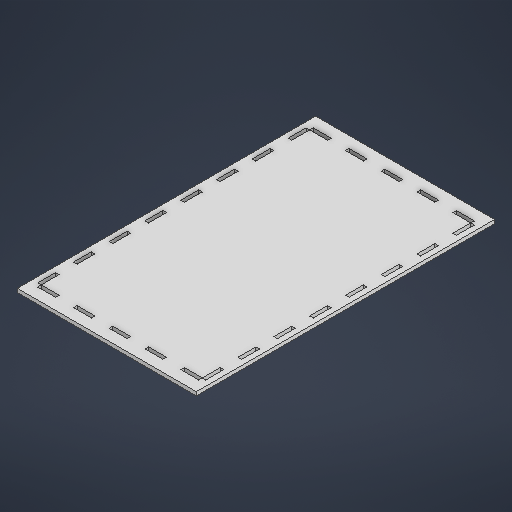
# Autodesk Inventor part: base
Saved by Autodesk Inventor 2026 (Build 300175000, 175)
## iProperties
Created: 2026-04-21
Part Number: base
Material: Generic
Document SubType Name: Modeling
Designer: juana
Density: 1 g/cm^3
Appearance: Default
Author: juana
Autodesk Inventor part; units mm, degrees
ref_plane "YZ Plane" through (0, 0, 0) normal (1, 0, 0) x (0, 1, 0)
ref_plane "XZ Plane" through (0, 0, 0) normal (0, 1, 0) x (-1, 0, 0)
ref_plane "XY Plane" through (0, 0, 0) normal (0, 0, 1) x (1, 0, 0)
sketch "Sketch1" plane through (0, 0, 0) normal (0, 1, 0) x (-1, 0, 0)
  line L0 (0, 0) -> (-150, 0)
  line L1 (-150, 0) -> (-150, -250)
  line L2 (-150, -250) -> (0, -250)
  line L3 (0, -250) -> (0, 0)
  dimension "d0" = 250
  dimension "d1" = 150
  constraints: 8 end point, 2 parallel, 1 coincident, 1 horizontal, 1 horizontal alignment, 1 perpendicular
  measures "d0" distance of L2.end L0.start
  measures "d1" distance of L0.start L0.end
extrude "Extrusion1" add sketch "Sketch1" along normal blind 3.05
sketch "Sketch2" plane through (0, 3.05, 0) normal (0, 1, 0) x (1, 0, 0)
  line L0 (7.5, 9.5) -> (22.5, 9.5)
  line L1 (22.5, 9.5) -> (22.5, 12.5)
  line L2 (22.5, 12.5) -> (7.5, 12.5)
  line L3 (7.5, 12.5) -> (7.5, 9.5)
  line L4 (7.5, 12.5) -> (142.5, 12.5) construction
  line L5 (142.5, 12.5) -> (142.5, 237.5) construction
  line L6 (142.5, 237.5) -> (7.5, 237.5) construction
  line L7 (7.5, 237.5) -> (7.5, 12.5) construction
  line L8 (0, 0) -> (150, 0) projected
  line L9 (0, 250) -> (0, 0) projected
  line L10 (37.5, 12.5) -> (37.5, 9.5)
  line L11 (37.5, 9.5) -> (52.5, 9.5)
  line L12 (52.5, 12.5) -> (37.5, 12.5)
  line L13 (52.5, 9.5) -> (52.5, 12.5)
  line L14 (67.5, 12.5) -> (67.5, 9.5)
  line L15 (67.5, 9.5) -> (82.5, 9.5)
  line L16 (82.5, 12.5) -> (67.5, 12.5)
  line L17 (82.5, 9.5) -> (82.5, 12.5)
  line L18 (97.5, 12.5) -> (97.5, 9.5)
  line L19 (97.5, 9.5) -> (112.5, 9.5)
  line L20 (112.5, 12.5) -> (97.5, 12.5)
  line L21 (112.5, 9.5) -> (112.5, 12.5)
  line L22 (127.5, 12.5) -> (127.5, 9.5)
  line L23 (127.5, 9.5) -> (142.5, 9.5)
  line L24 (142.5, 12.5) -> (127.5, 12.5)
  line L25 (142.5, 9.5) -> (142.5, 12.5)
  line L26 (7.5, 240.5) -> (7.5, 237.5)
  line L27 (7.5, 237.5) -> (22.5, 237.5)
  line L28 (22.5, 240.5) -> (7.5, 240.5)
  line L29 (22.5, 237.5) -> (22.5, 240.5)
  line L30 (37.5, 240.5) -> (37.5, 237.5)
  line L31 (37.5, 237.5) -> (52.5, 237.5)
  line L32 (52.5, 240.5) -> (37.5, 240.5)
  line L33 (52.5, 237.5) -> (52.5, 240.5)
  line L34 (67.5, 240.5) -> (67.5, 237.5)
  line L35 (67.5, 237.5) -> (82.5, 237.5)
  line L36 (82.5, 240.5) -> (67.5, 240.5)
  line L37 (82.5, 237.5) -> (82.5, 240.5)
  line L38 (97.5, 240.5) -> (97.5, 237.5)
  line L39 (97.5, 237.5) -> (112.5, 237.5)
  line L40 (112.5, 240.5) -> (97.5, 240.5)
  line L41 (112.5, 237.5) -> (112.5, 240.5)
  line L42 (127.5, 240.5) -> (127.5, 237.5)
  line L43 (127.5, 237.5) -> (142.5, 237.5)
  line L44 (142.5, 240.5) -> (127.5, 240.5)
  line L45 (142.5, 237.5) -> (142.5, 240.5)
  line L46 (142.5, 12.5) -> (145.5, 12.5)
  line L47 (145.5, 12.5) -> (145.5, 27.5)
  line L48 (145.5, 27.5) -> (142.5, 27.5)
  line L49 (142.5, 27.5) -> (142.5, 12.5)
  line L50 (142.5, 57.5) -> (142.5, 42.5)
  line L51 (142.5, 42.5) -> (145.5, 42.5)
  line L52 (145.5, 57.5) -> (142.5, 57.5)
  line L53 (145.5, 42.5) -> (145.5, 57.5)
  line L54 (142.5, 87.5) -> (142.5, 72.5)
  line L55 (142.5, 72.5) -> (145.5, 72.5)
  line L56 (145.5, 87.5) -> (142.5, 87.5)
  line L57 (145.5, 72.5) -> (145.5, 87.5)
  line L58 (142.5, 117.5) -> (142.5, 102.5)
  line L59 (142.5, 102.5) -> (145.5, 102.5)
  line L60 (145.5, 117.5) -> (142.5, 117.5)
  line L61 (145.5, 102.5) -> (145.5, 117.5)
  line L62 (142.5, 147.5) -> (142.5, 132.5)
  line L63 (142.5, 132.5) -> (145.5, 132.5)
  line L64 (145.5, 147.5) -> (142.5, 147.5)
  line L65 (145.5, 132.5) -> (145.5, 147.5)
  line L66 (142.5, 177.5) -> (142.5, 162.5)
  line L67 (142.5, 162.5) -> (145.5, 162.5)
  line L68 (145.5, 177.5) -> (142.5, 177.5)
  line L69 (145.5, 162.5) -> (145.5, 177.5)
  line L70 (142.5, 207.5) -> (142.5, 192.5)
  line L71 (142.5, 192.5) -> (145.5, 192.5)
  line L72 (145.5, 207.5) -> (142.5, 207.5)
  line L73 (145.5, 192.5) -> (145.5, 207.5)
  line L74 (142.5, 237.5) -> (142.5, 222.5)
  line L75 (142.5, 222.5) -> (145.5, 222.5)
  line L76 (145.5, 237.5) -> (142.5, 237.5)
  line L77 (145.5, 222.5) -> (145.5, 237.5)
  line L78 (4.5, 27.5) -> (4.5, 12.5)
  line L79 (4.5, 12.5) -> (7.5, 12.5)
  line L80 (7.5, 27.5) -> (4.5, 27.5)
  line L81 (7.5, 12.5) -> (7.5, 27.5)
  line L82 (4.5, 57.5) -> (4.5, 42.5)
  line L83 (4.5, 42.5) -> (7.5, 42.5)
  line L84 (7.5, 57.5) -> (4.5, 57.5)
  line L85 (7.5, 42.5) -> (7.5, 57.5)
  line L86 (4.5, 87.5) -> (4.5, 72.5)
  line L87 (4.5, 72.5) -> (7.5, 72.5)
  line L88 (7.5, 87.5) -> (4.5, 87.5)
  line L89 (7.5, 72.5) -> (7.5, 87.5)
  line L90 (4.5, 117.5) -> (4.5, 102.5)
  line L91 (4.5, 102.5) -> (7.5, 102.5)
  line L92 (7.5, 117.5) -> (4.5, 117.5)
  line L93 (7.5, 102.5) -> (7.5, 117.5)
  line L94 (4.5, 147.5) -> (4.5, 132.5)
  line L95 (4.5, 132.5) -> (7.5, 132.5)
  line L96 (7.5, 147.5) -> (4.5, 147.5)
  line L97 (7.5, 132.5) -> (7.5, 147.5)
  line L98 (4.5, 177.5) -> (4.5, 162.5)
  line L99 (4.5, 162.5) -> (7.5, 162.5)
  line L100 (7.5, 177.5) -> (4.5, 177.5)
  line L101 (7.5, 162.5) -> (7.5, 177.5)
  line L102 (4.5, 207.5) -> (4.5, 192.5)
  line L103 (4.5, 192.5) -> (7.5, 192.5)
  line L104 (7.5, 207.5) -> (4.5, 207.5)
  line L105 (7.5, 192.5) -> (7.5, 207.5)
  line L106 (4.5, 237.5) -> (4.5, 222.5)
  line L107 (4.5, 222.5) -> (7.5, 222.5)
  line L108 (7.5, 237.5) -> (4.5, 237.5)
  line L109 (7.5, 222.5) -> (7.5, 237.5)
  point P0 (75, 12.5)
  point P1 (75, 0)
  point P2 (7.5, 125)
  point P3 (0, 125)
  dimension "d4" = 3
  dimension "d5" = 15
  dimension "d6" = 225
  dimension "d7" = 135
  dimension "d11" = 30
  dimension "d14" = 228
  dimension "d19" = 3
  dimension "d20" = 15
  dimension "d31" = 30
  dimension "d34" = 138
  constraints: 216 end point, 6 parallel, 5 horizontal, 4 coincident, 4 midpoint, 3 perpendicular, 2 vertical, 1 horizontal alignment, 1 vertical alignment, 192 other
  measures "d4" distance of L2.end L0.start
  measures "d5" distance of L1.end L2.end
  measures "d6" distance of L6.end L4.start
  measures "d7" distance of L4.start L4.end
  measures "d11" distance of L2.end L10.start
  measures "d14" distance of L2.end L26.start
  measures "d19" distance of L48.end L47.end
  measures "d20" distance of L46.end L47.end
  measures "d31" distance of L48.end L50.start
  measures "d34" distance of L48.end L78.start
extrude "Extrusion2" cut sketch "Sketch2" against normal blind 228
equation "\"d17\" = d14"
body "Solid1"
